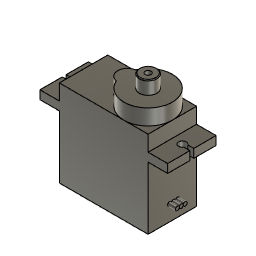
SG90_Micro Servo 9g v1 (Autodesk Fusion 360 design; units mm, degrees)
Autodesk Fusion 360 part; units mm, degrees
note: some values were not read from the file. Set by a fixed rule: which sketch regions a step uses.
sketch "alap" plane through (0, 0, 0) normal (0, 0, 1) x (1, 0, 0)
  line L0 (0, 0) -> (22.7, 0)
  line L1 (22.7, 0) -> (22.7, 12.4)
  line L2 (22.7, 12.4) -> (0, 12.4)
  line L3 (0, 12.4) -> (0, 0)
  dimension "d1" = 22.7
  dimension "d2" = 12.4
  constraint horizontal L0
  constraint vertical L1
  constraint horizontal L2
  constraint vertical L3
  constraint coincident L0.start L3.end
  measures "d1" distance of L0.start L0.end
  measures "d2" distance of L0.start L2.end
extrude "Extrude1" add sketch "alap" along normal blind 16 makes body 1
sketch "felso_alap" plane through (0, 0, 16) normal (0, 0, 1) x (-1, 0, 0)
  line L0 (0, 0) -> (-22.7, 0)
  line L1 (-22.7, -12.4) -> (0, -12.4)
  line L2 (0, 0) -> (-22.7, 0)
  line L3 (-22.7, 0) -> (-27.7, 0)
  line L4 (0, 0) -> (5, 0)
  line L5 (5, 0) -> (-22.7, 0)
  line L6 (-22.7, -12.4) -> (5, -12.4)
  line L7 (5, -12.4) -> (5, 0)
  line L8 (-27.7, 0) -> (-22.7, 0)
  line L9 (-22.7, -12.4) -> (-27.7, -12.4)
  line L10 (-27.7, -12.4) -> (-27.7, 0)
  dimension "d5" = 5
  dimension "d6" = 5
  constraint coincident L0.start L2.start
  constraint coincident L0.end L2.end
  constraint horizontal L5
  constraint horizontal L6
  constraint vertical L7
  constraint coincident L1.start L6.start
  constraint horizontal L8
  constraint horizontal L9
  constraint vertical L10
  measures "d5" distance of L0.end L3.end
  measures "d6" distance of L0.start L4.end
extrude "Extrude2" add sketch "felso_alap" along normal blind 2.2 bodies 1
sketch "felso_teto" plane through (0, 0, 18.2) normal (0, 0, 1) x (-1, 0, 0)
  line L0 (-27.7, -12.4) -> (5, -12.4)
  line L1 (5, -12.4) -> (5, 0)
  line L2 (5, 0) -> (-27.7, 0)
  line L3 (-27.7, 0) -> (-27.7, -12.4)
  line L4 (0.0248, -12.4) -> (-22.7, -12.4)
  line L5 (-22.7, -12.4) -> (-22.7, 0)
  line L6 (-22.7, 0) -> (0.0248, 0)
  line L7 (0.0248, 0) -> (0.0248, -12.4)
  constraint horizontal L4
  constraint vertical L5
  constraint horizontal L6
  constraint vertical L7
  constraint coincident L2 L5.end
  constraint coincident L0 L4.start
extrude "Extrude3" add sketch "felso_teto" along normal blind 4 separate body contours L0 L2 L4 L5 L6 L7 makes body 2
combine "Combine1" operation add target body 2 tool bodies 1
sketch "gear_haus" plane through (0, 0, 22.2) normal (0, 0, 1) x (-1, 0, 0)
  line L0 (0.0248, 0) -> (-22.7, 0)
  line L1 (-22.7, 0) -> (-22.7, -12.4)
  line L2 (-22.7, -12.4) -> (0.0248, -12.4)
  line L3 (0.0248, -12.4) -> (0.0248, 0)
  circle A0 centre (-16.5, -6.2) radius 6.2
  line L4 (-22.7, -6.2144) -> (-8.7, -6.2144) construction
  circle A1 centre (-11.2076, -6.2144) radius 2.5
  dimension "d11" = 12.4
  dimension "d14" = 14
  dimension "d16" = 5
  constraint coincident A0 L4.start
  constraint horizontal L4
  constraint coincident L4 A1.centre
  measures "d11" diameter of A0
  measures "d14" distance of L4.start L4.end
  measures "d16" diameter of A1
extrude "Extrude4" add sketch "gear_haus" along normal blind 4 contours A0 A1 | A0 A1 | A0 A1 bodies 2
sketch "Sketch7" plane through (0, 0, 26.2) normal (0, 0, 1) x (-1, 0, 0)
  arc A0 (-10.8194, -8.6841) -> (-10.806, -3.7469) centre (-11.2076, -6.2144) ccw
  arc A1 (-10.806, -3.7469) -> (-10.8194, -8.6841) centre (-16.5, -6.2) ccw
  circle A2 centre (-16.5, -6.2) radius 2.25
  dimension "d19" = 4.5
  measures "d19" diameter of A2
extrude "Extrude5" add sketch "Sketch7" along normal blind 3.4 contours A2 bodies 2
sketch "Sketch8" plane through (0, 0, 29.6) normal (0, 0, 1) x (-1, 0, 0)
  circle A0 centre (-16.5, -6.2) radius 2.25
  circle A1 centre (-16.5, -6.2) radius 0.75
  dimension "d22" = 1.5
  constraint concentric A0 A1
  measures "d22" diameter of A1
extrude "Extrude6" cut sketch "Sketch8" against normal blind 4 contours A1 bodies 2
fillet "Fillet1" radius 0.2 1 edges at (18.5977, 7.0136, 29.6) on bodies 2
sketch "Sketch10" plane through (0, 0, 18.2) normal (0, 0, 1) x (-1, 0, 0)
  line L0 (-22.7, -12.4) -> (-22.7, 0)
  line L1 (-22.7, 0) -> (-27.7, 0)
  line L2 (-27.7, 0) -> (-27.7, -12.4)
  line L3 (-27.7, -12.4) -> (-22.7, -12.4)
  line L4 (5.7217, -6.2) -> (-31, -6.2) construction
  line L5 (-25.3, -6.2) -> (-25.3, -6.7)
  line L6 (-25.3, -6.7) -> (-27.7, -6.7)
  line L7 (-27.7, -6.7) -> (-27.7, -6.2)
  line L8 (-25.3, -6.2) -> (-25.3, -5.7)
  line L9 (-25.3, -5.7) -> (-27.7, -5.7)
  line L10 (-27.7, -5.7) -> (-27.7, -6.2)
  circle A0 centre (-25.3, -6.2) radius 1
  line L11 (5.0007, -12.4) -> (-27.7, -12.4) construction
  line L12 (-11.3497, -12.4) -> (-11.3497, 3) construction
  circle A1 centre (2.6007, -6.2) radius 1
  line L13 (2.6007, -5.7) -> (5.0007, -5.7)
  line L14 (2.6007, -6.2) -> (2.6007, -5.7)
  line L15 (2.6007, -6.2) -> (2.6007, -6.7)
  line L16 (2.6007, -6.7) -> (5.0007, -6.7)
  line L17 (5.0007, -6.7) -> (5.0007, -5.7)
  dimension "d30" = 2.4
  dimension "d31" = 0.5
  dimension "d32" = 2
  constraint perpendicular L2 L4
  constraint vertical L5
  constraint horizontal L6
  constraint vertical L7
  constraint midpoint L2 L7.end
  constraint vertical L8
  constraint horizontal L9
  constraint vertical L10
  constraint coincident L5.start L8.start
  constraint coincident L2.end L3.start
  constraint perpendicular L2 L11
  constraint midpoint L11 L12.start
  constraint perpendicular L4 L12
  constraint symmetric L5.start L12 A1.centre
  constraint symmetric L5.end L12 L15.end
  constraint symmetric L6.end L12 L16.end
  constraint symmetric L8.end L12 L13.start
  constraint symmetric L9.end L12 L13.end
  constraint symmetric A0 L12 A1
  constraint perpendicular L13 L17
  measures "d30" distance of L7.end L5.start
  measures "d31" distance of L7.end L9.end
  measures "d32" diameter of A0
extrude "Extrude7" cut sketch "Sketch10" against normal blind 4 contours L2 L6 L7 L9 L10 A0 | L5 L6 L8 L9 A0 | L5 L6 L8 L9 A0 bodies 2
extrude "Extrude8" cut sketch "Sketch10" against normal blind 4 contours A1 L13 L14 L15 L16 | A1 L13 L16 L17 | A1 L13 L14 L15 L16 bodies 2
sketch "vezetek" plane through (22.7, 0, 0) normal (1, 0, 0) x (0, 1, 0)
  line L0 (0, 0) -> (12.4, 0)
  line L1 (12.4, 0) -> (12.4, 16)
  line L2 (12.4, 16) -> (0, 16)
  line L3 (0, 16) -> (0, 0)
  circle A0 centre (5.5, 4) radius 0.5
  circle A1 centre (6.5, 4) radius 0.5
  circle A2 centre (7.5, 4) radius 0.5
  line L4 (6.5, 0) -> (6.5, 4) construction
  line L5 (0, 4) -> (4, 4) construction
  dimension "d37" = 1
  dimension "d38" = 1
  dimension "d39" = 4
  dimension "d40" = 4
  constraint coincident L0 L4.start
  constraint perpendicular L0 L4
  constraint coincident L3 L5.start
  constraint perpendicular L3 L5
  measures "d37" diameter of A0
  measures "d38" diameter of A2
  measures "d39" distance of L4.start A1.centre
  measures "d40" distance of L5.start L5.end
extrude "Extrude9" add sketch "vezetek" along normal blind 2 separate body contours A0 | A2 | A1 makes body 3 at (24.0333, 7.6354, 4.4813)
named bodies: "towerPro SG90", "vezetek"
